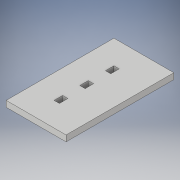
# Autodesk Inventor part: LEDFront
Saved by Autodesk Inventor 2019 (Build 230136000, 136)
## iProperties
Created: 2018-12-07
Part Number: LEDFront
Material: Generic
Document SubType Name: Modeling
Designer: Administrator
Density: 1 g/cm^3
Appearance: Default
Author: Administrator
Autodesk Inventor part; units mm, degrees
ref_plane "YZ Plane" through (0, 0, 0) normal (1, 0, 0) x (0, 1, 0)
ref_plane "XZ Plane" through (0, 0, 0) normal (0, 1, 0) x (-1, 0, 0)
ref_plane "XY Plane" through (0, 0, 0) normal (0, 0, 1) x (1, 0, 0)
sketch "Sketch1" plane through (0, 0, 0) normal (0, 1, 0) x (-1, 0, 0)
  line L0 (0, 0) -> (63.5, 0)
  line L1 (63.5, 0) -> (63.5, -114.3)
  line L2 (63.5, -114.3) -> (0, -114.3)
  line L3 (0, -114.3) -> (0, 0)
  line L4 (38.1, -52.6288) -> (32.4358, -52.6288)
  line L5 (32.4358, -52.6288) -> (32.4358, -61.6712)
  line L6 (32.4358, -61.6712) -> (38.1, -61.6712)
  line L7 (38.1, -61.6712) -> (38.1, -52.6288)
  line L8 (38.1, -25.4) -> (32.4358, -25.4)
  line L9 (32.4358, -25.4) -> (32.4358, -34.4424)
  line L10 (32.4358, -34.4424) -> (38.1, -34.4424)
  line L11 (38.1, -34.4424) -> (38.1, -25.4)
  line L12 (38.1, -79.8576) -> (32.4358, -79.8576)
  line L13 (32.4358, -79.8576) -> (32.4358, -88.9)
  line L14 (32.4358, -88.9) -> (38.1, -88.9)
  line L15 (38.1, -88.9) -> (38.1, -79.8576)
  dimension "d0" = 63.5
  dimension "d1" = 114.3
  dimension "d2" = 5.6642
  dimension "d3" = 9.0424
  dimension "d4" = 5.6642
  dimension "d5" = 9.0424
  dimension "d8" = 5.6642
  dimension "d9" = 9.0424
  dimension "d10" = 25.4
  dimension "d11" = 25.4
  dimension "d12" = 25.4
  dimension "d13" = 25.4
  dimension "d14" = 25.4
  dimension "d15" = 45.4152
  dimension "d16" = 18.1864
  dimension "d17" = 18.1864
  constraints: 32 end point, 8 parallel, 4 horizontal, 4 perpendicular
  measures "d0" distance of L1.end L2.end
  measures "d1" distance of L0.end L1.end
  measures "d2" distance of L6.end L5.end
  measures "d3" distance of L5.end L4.end
  measures "d4" distance of L10.end L9.end
  measures "d5" distance of L9.end L8.end
  measures "d8" distance of L14.end L13.end
  measures "d9" distance of L13.end L12.end
  measures "d10" distance between parallel lines of L1 L11
  measures "d11" distance between parallel lines of L7 L1
  measures "d12" distance between parallel lines of L1 L15
  measures "d13" distance between parallel lines of L2 L14
  measures "d14" distance between parallel lines of L0 L8
  measures "d15" distance between parallel lines of L12 L10
  measures "d16" distance between parallel lines of L10 L4
  measures "d17" distance between parallel lines of L12 L6
extrude "Extrusion1" add sketch "Sketch1" along normal blind 6.35
equation "\"d11\" = d10"
equation "\"d12\" = d11"
body "Solid1"
